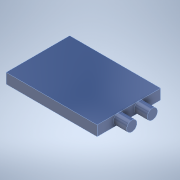
# Autodesk Inventor part: Lipo Battery
Saved by Autodesk Inventor 2021 (Build 250183000, 183)
## iProperties
Created: 2020-09-11
Part Number: Lipo Battery
Material: Generic
Document SubType Name: Modeling
Designer: jgray
Density: 1 g/cm^3
Appearance: Flaked Satin - Blue
Author: jgray
Autodesk Inventor part; units mm, degrees
ref_plane "YZ Plane" through (0, 0, 0) normal (1, 0, 0) x (0, 1, 0)
ref_plane "XZ Plane" through (0, 0, 0) normal (0, 1, 0) x (-1, 0, 0)
ref_plane "XY Plane" through (0, 0, 0) normal (0, 0, 1) x (1, 0, 0)
sketch "Sketch1" plane through (0, 0, 0) normal (0, 1, 0) x (-1, 0, 0)
  line L0 (0, 0) -> (62, 0)
  line L1 (62, 0) -> (62, -43.3)
  line L2 (62, -43.3) -> (0, -43.3)
  line L3 (0, -43.3) -> (0, 0)
  dimension "d0" = 62
  dimension "d1" = 43.3
  constraints: 8 end point, 2 parallel, 1 horizontal, 1 perpendicular
  measures "d0" distance of L1.end L2.end
  measures "d1" distance of L0.end L1.end
extrude "Extrusion1" add sketch "Sketch1" along normal blind 7
sketch "Sketch2" plane through (0, 0, 0) normal (1, 0, 0) x (0, 0, -1)
  line L0 (-9.6515, 3.5) -> (65.4292, 3.5) construction
  line L1 (0, 0) -> (0, 7) construction
  line L2 (21.65, 19.1254) -> (21.65, -18.6518) construction
  line L3 (0, 7) -> (43.3, 7) construction
  circle A0 centre (14.65, 3.5) radius 3.5
  circle A1 centre (28.65, 3.5) radius 3.5
  point P0 (0, 3.5)
  point P1 (21.65, 7)
  dimension "d4" = 7
  dimension "d5" = 7
  dimension "d6" = 14
  dimension "d7" = 7
  constraints: 4 end point, 4 point on line, 2 centre point, 2 midpoint, 1 horizontal, 1 vertical
  measures "d4" diameter of A0
  measures "d5" diameter of A1
  measures "d6" distance of A1.centre A0.centre
  measures "d7" distance from line of A1.centre L2
extrude "Extrusion2" add sketch "Sketch2" along normal blind 9
body "Solid1"
